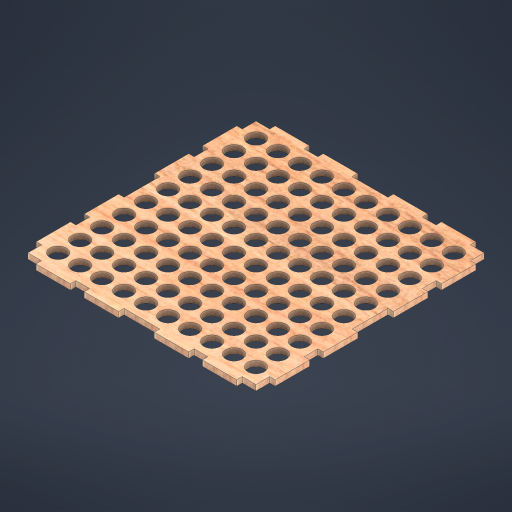
# Autodesk Inventor part: Middle
Saved by Autodesk Inventor 2024.1 (Build 281209000, 209)
## iProperties
Created: 2024-05-23
Part Number: Middle
Material: Wood (Birch)
Document SubType Name: Modeling
Designer: Tim Jäger
Density: 0.55 g/cm^3
Appearance: Birch - Natural Polished
Author: Tim Jäger
Autodesk Inventor part; units mm, degrees
ref_plane "YZ Plane" through (0, 0, 0) normal (1, 0, 0) x (0, 1, 0)
ref_plane "XZ Plane" through (0, 0, 0) normal (0, 1, 0) x (-1, 0, 0)
ref_plane "XY Plane" through (0, 0, 0) normal (0, 0, 1) x (1, 0, 0)
sketch "Sketch1" plane through (0, 0, 0) normal (0, 1, 0) x (-1, 0, 0)
  line L0 (-83, 83) -> (83, 83)
  line L1 (83, 83) -> (83, -83)
  line L2 (83, -83) -> (-83, -83)
  line L3 (-83, -83) -> (-83, 83)
  line L4 (-83, 83) -> (83, -83) construction
  line L5 (83, 83) -> (-83, -83) construction
  circle A0 centre (72, -72) radius 6
  circle A1 centre (56, -72) radius 6
  circle A2 centre (40, -72) radius 6
  circle A3 centre (24, -72) radius 6
  circle A4 centre (8, -72) radius 6
  circle A5 centre (-8, -72) radius 6
  circle A6 centre (-24, -72) radius 6
  circle A7 centre (-40, -72) radius 6
  circle A8 centre (-56, -72) radius 6
  circle A9 centre (-72, -72) radius 6
  circle A10 centre (72, -56) radius 6
  circle A11 centre (56, -56) radius 6
  circle A12 centre (40, -56) radius 6
  circle A13 centre (24, -56) radius 6
  circle A14 centre (8, -56) radius 6
  circle A15 centre (-8, -56) radius 6
  circle A16 centre (-24, -56) radius 6
  circle A17 centre (-40, -56) radius 6
  circle A18 centre (-56, -56) radius 6
  circle A19 centre (-72, -56) radius 6
  circle A20 centre (72, -40) radius 6
  circle A21 centre (56, -40) radius 6
  circle A22 centre (40, -40) radius 6
  circle A23 centre (24, -40) radius 6
  circle A24 centre (8, -40) radius 6
  circle A25 centre (-8, -40) radius 6
  circle A26 centre (-24, -40) radius 6
  circle A27 centre (-40, -40) radius 6
  circle A28 centre (-56, -40) radius 6
  circle A29 centre (-72, -40) radius 6
  circle A30 centre (72, -24) radius 6
  circle A31 centre (56, -24) radius 6
  circle A32 centre (40, -24) radius 6
  circle A33 centre (24, -24) radius 6
  circle A34 centre (8, -24) radius 6
  circle A35 centre (-8, -24) radius 6
  circle A36 centre (-24, -24) radius 6
  circle A37 centre (-40, -24) radius 6
  circle A38 centre (-56, -24) radius 6
  circle A39 centre (-72, -24) radius 6
  circle A40 centre (72, -8) radius 6
  circle A41 centre (56, -8) radius 6
  circle A42 centre (40, -8) radius 6
  circle A43 centre (24, -8) radius 6
  circle A44 centre (8, -8) radius 6
  circle A45 centre (-8, -8) radius 6
  circle A46 centre (-24, -8) radius 6
  circle A47 centre (-40, -8) radius 6
  circle A48 centre (-56, -8) radius 6
  circle A49 centre (-72, -8) radius 6
  circle A50 centre (72, 8) radius 6
  circle A51 centre (56, 8) radius 6
  circle A52 centre (40, 8) radius 6
  circle A53 centre (24, 8) radius 6
  circle A54 centre (8, 8) radius 6
  circle A55 centre (-8, 8) radius 6
  circle A56 centre (-24, 8) radius 6
  circle A57 centre (-40, 8) radius 6
  circle A58 centre (-56, 8) radius 6
  circle A59 centre (-72, 8) radius 6
  circle A60 centre (72, 24) radius 6
  circle A61 centre (56, 24) radius 6
  circle A62 centre (40, 24) radius 6
  circle A63 centre (24, 24) radius 6
  circle A64 centre (8, 24) radius 6
  circle A65 centre (-8, 24) radius 6
  circle A66 centre (-24, 24) radius 6
  circle A67 centre (-40, 24) radius 6
  circle A68 centre (-56, 24) radius 6
  circle A69 centre (-72, 24) radius 6
  circle A70 centre (72, 40) radius 6
  circle A71 centre (56, 40) radius 6
  circle A72 centre (40, 40) radius 6
  circle A73 centre (24, 40) radius 6
  circle A74 centre (8, 40) radius 6
  circle A75 centre (-8, 40) radius 6
  circle A76 centre (-24, 40) radius 6
  circle A77 centre (-40, 40) radius 6
  circle A78 centre (-56, 40) radius 6
  circle A79 centre (-72, 40) radius 6
  circle A80 centre (72, 56) radius 6
  circle A81 centre (56, 56) radius 6
  circle A82 centre (40, 56) radius 6
  circle A83 centre (24, 56) radius 6
  circle A84 centre (8, 56) radius 6
  circle A85 centre (-8, 56) radius 6
  circle A86 centre (-24, 56) radius 6
  circle A87 centre (-40, 56) radius 6
  circle A88 centre (-56, 56) radius 6
  circle A89 centre (-72, 56) radius 6
  circle A90 centre (72, 72) radius 6
  circle A91 centre (56, 72) radius 6
  circle A92 centre (40, 72) radius 6
  circle A93 centre (24, 72) radius 6
  circle A94 centre (8, 72) radius 6
  circle A95 centre (-8, 72) radius 6
  circle A96 centre (-24, 72) radius 6
  circle A97 centre (-40, 72) radius 6
  circle A98 centre (-56, 72) radius 6
  circle A99 centre (-72, 72) radius 6
  line L6 (72, -72) -> (-72, 72) construction
  line L7 (83, -73) -> (87, -73)
  line L8 (87, -73) -> (87, -48)
  line L9 (87, -48) -> (83, -48)
  line L10 (83, -48) -> (83, -73)
  line L11 (73, -83) -> (48, -83)
  line L12 (48, -83) -> (48, -87)
  line L13 (48, -87) -> (73, -87)
  line L14 (73, -87) -> (73, -83)
  line L15 (83, -38) -> (87, -38)
  line L16 (87, -38) -> (87, -13)
  line L17 (87, -13) -> (83, -13)
  line L18 (83, -13) -> (83, -38)
  line L19 (38, -83) -> (13, -83)
  line L20 (13, -83) -> (13, -87)
  line L21 (13, -87) -> (38, -87)
  line L22 (38, -87) -> (38, -83)
  line L23 (73, 83) -> (73, 87)
  line L24 (13, 87) -> (13, 83)
  line L25 (13, 83) -> (38, 83)
  line L26 (38, 83) -> (38, 87)
  line L27 (48, 87) -> (48, 83)
  line L28 (48, 83) -> (73, 83)
  line L29 (73, 87) -> (48, 87)
  line L30 (38, 87) -> (13, 87)
  line L31 (83, 73) -> (83, 48)
  line L32 (87, 73) -> (83, 73)
  line L33 (87, 48) -> (87, 73)
  line L34 (83, 48) -> (87, 48)
  line L35 (87, 38) -> (83, 38)
  line L36 (83, 13) -> (87, 13)
  line L37 (87, 13) -> (87, 38)
  line L38 (83, 38) -> (83, 13)
  line L39 (-83, 73) -> (-87, 73)
  line L40 (-87, 13) -> (-83, 13)
  line L41 (-83, 13) -> (-83, 38)
  line L42 (-83, 38) -> (-87, 38)
  line L43 (-87, 48) -> (-83, 48)
  line L44 (-83, 48) -> (-83, 73)
  line L45 (-87, 73) -> (-87, 48)
  line L46 (-87, 38) -> (-87, 13)
  line L47 (-73, 83) -> (-48, 83)
  line L48 (-73, 87) -> (-73, 83)
  line L49 (-48, 87) -> (-73, 87)
  line L50 (-48, 83) -> (-48, 87)
  line L51 (-38, 87) -> (-38, 83)
  line L52 (-13, 83) -> (-13, 87)
  line L53 (-13, 87) -> (-38, 87)
  line L54 (-38, 83) -> (-13, 83)
  line L55 (-73, -83) -> (-73, -87)
  line L56 (-13, -87) -> (-13, -83)
  line L57 (-13, -83) -> (-38, -83)
  line L58 (-38, -83) -> (-38, -87)
  line L59 (-48, -87) -> (-48, -83)
  line L60 (-48, -83) -> (-73, -83)
  line L61 (-73, -87) -> (-48, -87)
  line L62 (-38, -87) -> (-13, -87)
  line L63 (-83, -73) -> (-83, -48)
  line L64 (-87, -73) -> (-83, -73)
  line L65 (-87, -48) -> (-87, -73)
  line L66 (-83, -48) -> (-87, -48)
  line L67 (-87, -38) -> (-83, -38)
  line L68 (-83, -13) -> (-87, -13)
  line L69 (-87, -13) -> (-87, -38)
  line L70 (-83, -38) -> (-83, -13)
  point P0 (0, 0)
  point P1 (73, -85)
  point P2 (85, -38)
  point P3 (85, -48)
  point P4 (48, -85)
  point P5 (38, -85)
  point P6 (83, 83)
  point P7 (38, 85)
  point P8 (48, 85)
  point P9 (85, 73)
  point P10 (85, 48)
  point P11 (85, 38)
  point P12 (-83, 83)
  point P13 (-85, 38)
  point P14 (-85, 48)
  point P15 (-73, 85)
  point P16 (-48, 85)
  point P17 (-38, 85)
  point P18 (-38, -85)
  point P19 (-48, -85)
  point P20 (-85, -73)
  point P21 (-85, -48)
  point P22 (-85, -38)
  point P23 (-38, -83)
  dimension "d0" = 12
  dimension "d3" = 16
  dimension "d6" = 16
  dimension "d9" = 5
  dimension "d10" = 5
  dimension "d11" = 4
  dimension "d12" = 4
  dimension "d13" = 10
  dimension "d14" = 10
  dimension "d15" = 25
  dimension "d16" = 4
  dimension "d17" = 25
  dimension "d18" = 10
  dimension "d19" = 25
  dimension "d20" = 10
  dimension "d21" = 25
  dimension "d22" = 4
  dimension "d25" = 360
  constraints: 142 end point, 100 centre point, 10 parallel, 8 midpoint, 6 horizontal, 5 perpendicular, 4 point on line, 1 vertical, 351 other
  measures "d0" diameter of A0
  measures "d3" distance of L6.start A1.centre
  measures "d6" distance of L6.start A10.centre
  measures "d9" distance edge to line of A9 L3
  measures "d10" distance edge to line of A9 L2
  measures "d11" distance of L13.end L11.start
  measures "d12" distance of L7.start L7.end
  measures "d13" horizontal distance of L1.end point (73, -85)
  measures "d14" vertical distance of L1.end L7.end
  measures "d15" distance of L7.end L8.end
  measures "d16" distance of L17.end L16.end
  measures "d17" distance of L15.end L16.end
  measures "d18" distance of point (85, -38) point (85, -48)
  measures "d19" distance of L12.end L13.end
  measures "d20" distance of point (48, -85) point (38, -85)
  measures "d21" distance of L20.end L21.end
  measures "d22" distance between parallel lines of L2 L21
extrude "Extrusion1" add sketch "Sketch1" along normal blind 4
body "Solid1"
